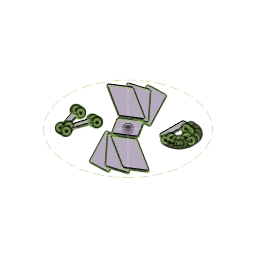
logo_for_modelling_join (Autodesk Fusion 360 design; units mm, degrees)
part number: 2026-05-07-17-58-11-378
part number: 2026-05-07-17-58-56-175
Autodesk Fusion 360 part; units mm, degrees
sketch "Sketch1" plane through (0, 0, 0) normal (0, 0, 1) x (1, 0, 0) in component "logo_nakres"
  line L0 (24.5875, 24.5875) -> (-24.5875, 24.5875) construction
  line L1 (-24.5875, 24.5875) -> (-24.5875, -24.5875) construction
  line L2 (-24.5875, -24.5875) -> (24.5875, -24.5875) construction
  line L3 (24.5875, -24.5875) -> (24.5875, 24.5875) construction
  line L4 (24.5875, 24.5875) -> (-24.5875, -24.5875) construction
  line L5 (-24.5875, 24.5875) -> (24.5875, -24.5875) construction
  line L6 (-4.5418, 19.8462) -> (-10.9856, 19.5937)
  arc A0 (-11.3602, 18.9462) -> (-10.9856, 19.5937) centre (-10.9683, 19.1516) cw
  arc A1 (3.4798, 5.9) -> (3.1052, 5.2525) centre (3.0879, 5.6946) cw
  line L7 (3.4798, 5.9) -> (-3.5173, 19.2535)
  arc A2 (-4.5418, 19.8462) -> (-3.5173, 19.2535) centre (-4.4984, 18.7394) cw
  line L8 (4.541, -19.8455) -> (10.9849, -19.5931)
  arc A3 (11.3595, -18.9456) -> (10.9849, -19.5931) centre (10.9676, -19.151) cw
  line L9 (11.3595, -18.9456) -> (10.6736, -17.6367)
  arc A4 (-3.4806, -5.8993) -> (-3.106, -5.2519) centre (-3.0886, -5.694) cw
  line L10 (-3.4806, -5.8993) -> (3.5166, -19.2529)
  arc A5 (4.541, -19.8455) -> (3.5166, -19.2528) centre (4.4976, -18.7388) cw
  circle A6 centre (-0.0004, 0.0003) radius 24.5875 construction
  line L11 (-9.5235, 17.9945) -> (-15.6825, 16.0829)
  arc A7 (-15.8767, 15.3605) -> (-15.6825, 16.0829) centre (-15.5513, 15.6603) cw
  line L12 (-15.8767, 15.3605) -> (-14.8755, 14.2737)
  arc A8 (1.8343, 6.5997) -> (1.64, 5.8773) centre (1.5089, 6.2999) cw
  line L13 (1.8343, 6.5997) -> (-8.3806, 17.6872)
  arc A9 (-9.5235, 17.9945) -> (-8.3806, 17.6872) centre (-9.1952, 16.9367) cw
  line L14 (9.5227, -17.9939) -> (15.6817, -16.0822)
  arc A10 (15.876, -15.3599) -> (15.6817, -16.0822) centre (15.5505, -15.6597) cw
  line L15 (15.876, -15.3599) -> (14.8747, -14.2731)
  arc A11 (-1.835, -6.599) -> (-1.6408, -5.8767) centre (-1.5096, -6.2992) cw
  line L16 (-1.835, -6.599) -> (8.3798, -17.6866)
  arc A12 (9.5227, -17.9939) -> (8.3798, -17.6866) centre (9.1944, -16.9361) cw
  line L17 (-13.8562, 14.9166) -> (-19.3106, 11.4761)
  arc A13 (-19.3113, 10.728) -> (-19.3106, 11.4761) centre (-19.0745, 11.1018) cw
  line L18 (-19.3113, 10.728) -> (-6.5748, 2.6621)
  arc A14 (-5.3913, 2.661) -> (-6.5748, 2.6621) centre (-5.9822, 3.5978) cw
  line L19 (-5.3913, 2.661) -> (0.063, 6.1016)
  arc A15 (0.0637, 6.8496) -> (0.063, 6.1016) centre (-0.173, 6.4758) cw
  line L20 (0.0637, 6.8496) -> (-12.6727, 14.9156)
  arc A16 (-13.8562, 14.9166) -> (-12.6727, 14.9156) centre (-13.2653, 13.9798) cw
  line L21 (1.5056, 4.8864) -> (4.9966, -0.6478)
  arc A17 (4.9966, -0.6478) -> (4.778, -1.6134) centre (4.4045, -1.0213) cw
  line L22 (4.778, -1.6134) -> (-0.7562, -5.1043)
  arc A18 (-0.7562, -5.1043) -> (-1.7218, -4.8857) centre (-1.1297, -4.5122) cw
  line L23 (-1.7218, -4.8857) -> (-5.2127, 0.6485)
  arc A19 (-5.2127, 0.6485) -> (-4.9941, 1.614) centre (-4.6206, 1.0219) cw
  line L24 (-4.9941, 1.614) -> (0.54, 5.105)
  arc A20 (0.54, 5.105) -> (1.5056, 4.8864) centre (0.9135, 4.5129) cw
  line L25 (13.8555, -14.916) -> (19.3098, -11.4754)
  arc A21 (19.3105, -10.7274) -> (19.3098, -11.4754) centre (19.0738, -11.1012) cw
  line L26 (19.3105, -10.7274) -> (6.5741, -2.6615)
  arc A22 (5.3905, -2.6604) -> (6.5741, -2.6615) centre (5.9815, -3.5972) cw
  line L27 (5.3905, -2.6604) -> (-0.0638, -6.101)
  arc A23 (-0.0645, -6.849) -> (-0.0638, -6.101) centre (0.1723, -6.4752) cw
  line L28 (-0.0645, -6.849) -> (12.672, -14.9149)
  arc A24 (13.8555, -14.916) -> (12.672, -14.9149) centre (13.2646, -13.9792) cw
  spline S0 degree 3 poles (-13.2277, -11.2522) (-13.1362, -11.6276) (-13.0465, -11.6278) (-12.9655, -11.2498) knots 0 0 0 0 1 1 1 1
  line L29 (-13.2277, -11.2522) -> (-13.1362, -11.6276) construction
  line L30 (-13.1362, -11.6276) -> (-13.0465, -11.6278) construction
  line L31 (-13.0465, -11.6278) -> (-12.9655, -11.2498) construction
  spline S1 degree 3 poles (17.197, 8.2576) (17.1492, 7.6922) (17.0411, 7.1804) (16.8728, 6.7224) knots 0 0 0 0 1 1 1 1
  line L32 (17.197, 8.2576) -> (17.1492, 7.6922) construction
  line L33 (17.1492, 7.6922) -> (17.0411, 7.1804) construction
  line L34 (17.0411, 7.1804) -> (16.8728, 6.7224) construction
  spline S2 degree 3 poles (16.8728, 6.7224) (16.7396, 6.3599) (16.4328, 5.8079) (16.1925, 5.5055) knots 0 0 0 0 1 1 1 1
  line L35 (16.8728, 6.7224) -> (16.7396, 6.3599) construction
  line L36 (16.7396, 6.3599) -> (16.4328, 5.8079) construction
  line L37 (16.4328, 5.8079) -> (16.1925, 5.5055) construction
  spline S3 degree 3 poles (16.1925, 5.5055) (15.9529, 5.2041) (15.6766, 4.9424) (15.3633, 4.7204) knots 0 0 0 0 1 1 1 1
  line L38 (16.1925, 5.5055) -> (15.9529, 5.2041) construction
  line L39 (15.9529, 5.2041) -> (15.6766, 4.9424) construction
  line L40 (15.6766, 4.9424) -> (15.3633, 4.7204) construction
  spline S4 degree 3 poles (15.3633, 4.7204) (15.0482, 4.4971) (14.4799, 4.2227) (14.1129, 4.1024) knots 0 0 0 0 1 1 1 1
  line L41 (15.3633, 4.7204) -> (15.0482, 4.4971) construction
  line L42 (15.0482, 4.4971) -> (14.4799, 4.2227) construction
  line L43 (14.4799, 4.2227) -> (14.1129, 4.1024) construction
  spline S5 degree 3 poles (14.1129, 4.1024) (13.6715, 3.9576) (13.192, 3.8633) (12.6744, 3.8193) knots 0 0 0 0 1 1 1 1
  line L44 (14.1129, 4.1024) -> (13.6715, 3.9576) construction
  line L45 (13.6715, 3.9576) -> (13.192, 3.8633) construction
  line L46 (13.192, 3.8633) -> (12.6744, 3.8193) construction
  spline S6 degree 3 poles (12.6744, 3.8193) (12.2893, 3.7866) (11.6618, 3.7905) (11.2751, 3.7905) knots 0 0 0 0 1 1 1 1
  line L47 (12.6744, 3.8193) -> (12.2893, 3.7866) construction
  line L48 (12.2893, 3.7866) -> (11.6618, 3.7905) construction
  line L49 (11.6618, 3.7905) -> (11.2751, 3.7905) construction
  line L50 (11.2751, 3.7905) -> (9.623, 3.7905)
  arc A25 (9.623, 3.7905) -> (8.923, 4.4906) centre (9.623, 4.4906) cw
  line L51 (8.923, 4.4906) -> (8.923, 13.0871)
  arc A26 (8.923, 13.0871) -> (9.623, 13.7871) centre (9.623, 13.0871) cw
  line L52 (9.623, 13.7871) -> (11.5272, 13.7871)
  spline S7 degree 3 poles (11.5272, 13.7871) (11.9138, 13.7871) (12.5414, 13.7913) (12.9264, 13.7577) knots 0 0 0 0 1 1 1 1
  line L53 (11.5272, 13.7871) -> (11.9138, 13.7871) construction
  line L54 (11.9138, 13.7871) -> (12.5414, 13.7913) construction
  line L55 (12.5414, 13.7913) -> (12.9264, 13.7577) construction
  spline S8 degree 3 poles (12.9264, 13.7577) (13.8809, 13.6742) (14.6881, 13.4137) (15.3481, 12.9761) knots 0 0 0 0 1 1 1 1
  line L56 (12.9264, 13.7577) -> (13.8809, 13.6742) construction
  line L57 (13.8809, 13.6742) -> (14.6881, 13.4137) construction
  line L58 (14.6881, 13.4137) -> (15.3481, 12.9761) construction
  spline S9 degree 3 poles (15.3481, 12.9761) (15.6699, 12.7628) (16.1323, 12.3308) (16.3618, 12.0204) knots 0 0 0 0 1 1 1 1
  line L59 (15.3481, 12.9761) -> (15.6699, 12.7628) construction
  line L60 (15.6699, 12.7628) -> (16.1323, 12.3308) construction
  line L61 (16.1323, 12.3308) -> (16.3618, 12.0204) construction
  spline S10 degree 3 poles (16.3618, 12.0204) (16.8274, 11.3907) (17.1047, 10.6026) (17.1939, 9.6559) knots 0 0 0 0 1 1 1 1
  line L62 (16.3618, 12.0204) -> (16.8274, 11.3907) construction
  line L63 (16.8274, 11.3907) -> (17.1047, 10.6026) construction
  line L64 (17.1047, 10.6026) -> (17.1939, 9.6559) construction
  spline S11 degree 3 poles (17.1939, 9.6559) (17.2301, 9.2711) (17.2296, 8.6427) (17.197, 8.2576) knots 0 0 0 0 1 1 1 1
  line L65 (17.1939, 9.6559) -> (17.2301, 9.2711) construction
  line L66 (17.2301, 9.2711) -> (17.2296, 8.6427) construction
  line L67 (17.2296, 8.6427) -> (17.197, 8.2576) construction
  spline S12 degree 3 poles (14.9473, 9.5715) (14.8981, 9.9944) (14.8011, 10.3612) (14.6563, 10.6718) knots 0 0 0 0 1 1 1 1
  line L68 (14.9473, 9.5715) -> (14.8981, 9.9944) construction
  line L69 (14.8981, 9.9944) -> (14.8011, 10.3612) construction
  line L70 (14.8011, 10.3612) -> (14.6563, 10.6718) construction
  spline S13 degree 3 poles (14.6563, 10.6718) (14.4936, 11.0207) (14.061, 11.4979) (13.7252, 11.686) knots 0 0 0 0 1 1 1 1
  line L71 (14.6563, 10.6718) -> (14.4936, 11.0207) construction
  line L72 (14.4936, 11.0207) -> (14.061, 11.4979) construction
  line L73 (14.061, 11.4979) -> (13.7252, 11.686) construction
  spline S14 degree 3 poles (13.7252, 11.686) (13.4753, 11.826) (13.1896, 11.9241) (12.868, 11.9803) knots 0 0 0 0 1 1 1 1
  line L74 (13.7252, 11.686) -> (13.4753, 11.826) construction
  line L75 (13.4753, 11.826) -> (13.1896, 11.9241) construction
  line L76 (13.1896, 11.9241) -> (12.868, 11.9803) construction
  spline S15 degree 3 poles (12.868, 11.9803) (12.4877, 12.0469) (11.8578, 12.037) (11.4712, 12.037) knots 0 0 0 0 1 1 1 1
  line L77 (12.868, 11.9803) -> (12.4877, 12.0469) construction
  line L78 (12.4877, 12.0469) -> (11.8578, 12.037) construction
  line L79 (11.8578, 12.037) -> (11.4712, 12.037) construction
  arc A27 (11.0651, 11.337) -> (11.4712, 12.037) centre (11.6182, 11.484) cw
  line L80 (11.0651, 11.337) -> (11.0651, 6.2547)
  arc A28 (11.7652, 5.5546) -> (11.0651, 6.2547) centre (11.7652, 6.2547) cw
  spline S16 degree 3 poles (11.7652, 5.5546) (11.8734, 5.5546) (12.277, 5.5461) (12.6587, 5.6047) knots 0 0 0 0 1 1 1 1
  line L81 (11.7652, 5.5546) -> (11.8734, 5.5546) construction
  line L82 (11.8734, 5.5546) -> (12.277, 5.5461) construction
  line L83 (12.277, 5.5461) -> (12.6587, 5.6047) construction
  spline S17 degree 3 poles (12.6587, 5.6047) (14.0127, 5.8129) (14.7757, 6.6693) (14.9478, 8.1742) knots 0 0 0 0 1 1 1 1
  line L84 (12.6587, 5.6047) -> (14.0127, 5.8129) construction
  line L85 (14.0127, 5.8129) -> (14.7757, 6.6693) construction
  line L86 (14.7757, 6.6693) -> (14.9478, 8.1742) construction
  spline S18 degree 3 poles (14.9478, 8.1742) (14.9917, 8.5581) (14.992, 9.1876) (14.9473, 9.5715) knots 0 0 0 0 1 1 1 1
  line L87 (14.9478, 8.1742) -> (14.9917, 8.5581) construction
  line L88 (14.9917, 8.5581) -> (14.992, 9.1876) construction
  line L89 (14.992, 9.1876) -> (14.9473, 9.5715) construction
  line L90 (-2.1647, 4.6964) -> (1.64, 5.8773)
  line L91 (-11.3602, 18.9462) -> (-10.6744, 17.6373)
  line L92 (1.1394, 5.1755) -> (3.1052, 5.2525)
  line L93 (-0.8755, 5.0965) -> (0.6365, 5.1558)
  line L94 (2.1639, -4.6958) -> (-1.6408, -5.8767)
  line L95 (-1.3322, -5.1824) -> (-3.106, -5.2519)
  line L96 (0.8747, -5.0959) -> (-0.8754, -5.1645)
  line L97 (-13.9029, -13.2982) -> (-12.2928, -13.2976) construction
  line L98 (-12.2928, -13.2976) -> (-8.8906, -4.0406) construction
  line L99 (-8.8906, -4.0406) -> (-10.3327, -4.2683) construction
  line L100 (-17.2049, -4.2765) -> (-17.2912, -4.0408) construction
  line L101 (-17.2912, -4.0408) -> (-15.8491, -4.2672) construction
  line L102 (-13.9029, -13.7865) -> (-12.2928, -13.7865)
  arc A29 (-14.3674, -13.4489) -> (-13.9029, -13.7865) centre (-13.9029, -13.2983) ccw
  line L103 (-14.3674, -13.4489) -> (-17.5288, -4.1214)
  line L104 (-17.2913, -3.7899) -> (-15.8493, -3.7892)
  line L105 (-15.3924, -4.1278) -> (-13.2277, -11.2522)
  line L106 (-12.9655, -11.2498) -> (-10.7903, -4.1285)
  line L107 (-10.3329, -3.7898) -> (-8.8908, -3.7892)
  line L108 (-8.6536, -4.1204) -> (-11.8301, -13.4552)
  arc A30 (-10.3329, -3.7898) -> (-10.7903, -4.1285) centre (-10.3327, -4.2683) ccw
  line L109 (-13.9029, -13.2982) -> (-17.2049, -4.2765) construction
  arc A31 (-8.6536, -4.1204) -> (-8.8908, -3.7892) centre (-8.8907, -4.0397) ccw
  arc A32 (-12.2928, -13.7865) -> (-11.8301, -13.4552) centre (-12.2928, -13.2977) ccw
  arc A33 (-15.3924, -4.1278) -> (-15.8493, -3.7892) centre (-15.8491, -4.2665) ccw
  arc A34 (-17.2913, -3.7899) -> (-17.5288, -4.1214) centre (-17.2912, -4.0408) ccw
  point P0 (24.5871, 0.0003)
  dimension "d1" = 49.175
  dimension "d2" = 49.175
  constraint horizontal L0
  constraint perpendicular L0 L1
  constraint parallel L0 L2
  constraint parallel L1 L3
  constraint coincident L4 origin
  constraint coincident L5 origin
  constraint coincident L17 L12.end
  constraint coincident L19 L90.start
  constraint coincident L11 L91.end
  constraint coincident L90 L93.start
  constraint coincident A20 L93.end
  constraint coincident A20 L92.start
  constraint coincident L25 L15.end
  constraint coincident L27 L94.start
  constraint coincident A18 L95.start
  constraint coincident L94 L96.start
  constraint coincident A18 L96.end
  constraint coincident L14 L9.end
  constraint horizontal L102
  constraint tangent L102 A32
  constraint tangent L103 A34
  constraint tangent L104 A33
  constraint tangent L104 A34
  constraint coincident S0.start L29.start
  constraint tangent L105 A33
  constraint coincident S0.end L31.end
  constraint tangent L106 A30
  constraint tangent L107 A31
  constraint tangent L107 A30
  constraint tangent L108 A32
  constraint tangent L108 A31
  constraint coincident L100.start A34
  measures "d1" distance of L0.end L1.end
  measures "d2" distance of L1.end L2.end
extrude "Extrude1" add sketch "Sketch1" along normal blind 0.6 contours L21 A17 L22 A18 L23 A19 L24 A20 | L17 A13 L18 A14 L19 A15 L20 A16 | L25 A21 L26 A22 L27 A23 L28 A24 | S0 L102 A29 L103 L104 L105 L106 L107 L108 A30 A31 A32 A33 A34 | S1 S2 S3 S4 S5 S6 L50 A25 L51 A26 L52 S7 S8 S9 S10 S11 makes body 1 at (9.637, 7.9441, 0) makes body 2 at (0.3569, 1.3071, 0.6) makes body 3 at (-6.3946, 8.1424, 0) makes body 4 at (-11.1497, -9.6085, 0) makes body 5 at (6.3938, -8.1418, 0) in component "logo_nakres"
extrude "Extrude2" add sketch "Sketch1" along normal blind 0.4 contours L11 A7 L12 A8 L13 A9 L17 L19 A15 L20 A16 L90 | L14 A10 L15 A11 L16 A12 L25 L27 A23 L28 A24 L94 bodies 3 5 in component "logo_nakres"
extrude "Extrude3" add sketch "Sketch1" along normal blind 0.2 contours L6 A0 A1 L7 A2 L11 A8 L13 A9 A20 L90 L91 L92 L93 | L8 A3 L9 A4 L10 A5 L14 A11 L16 A12 A18 L94 L95 L96 bodies 2 3 5 in component "logo_nakres"
component "logo_nakres" placed x (1, 0, 0) y (0, 1, 0) z (0, 0, 1) at (0, 0, 0)
equation "d2 = d1"
equation "d3 = 3 * stupen_extrude"
equation "d5 = 2 * stupen_extrude"
equation "d7 = stupen_extrude"
equation "stupen_extrude = 0.2 mm"
